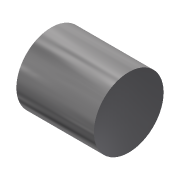
# Autodesk Inventor part: おもり
Saved by Autodesk Inventor 2013 (Build 170138000, 138)
## iProperties
Created: 2013-12-16
Part Number: おもり
Material: ステンレス鋼
Document SubType Name: Modeling
Designer: victor
Mass: 642.534 g
Surface Area: 102.494 cm^2
Volume: 79.5216 cm^3
Density: 8.08 g/cm^3
Author: victor
Autodesk Inventor part; units mm, degrees
ref_plane "YZ Plane" through (0, 0, 0) normal (1, 0, 0) x (0, 1, 0)
ref_plane "XZ Plane" through (0, 0, 0) normal (0, 1, 0) x (-1, 0, 0)
ref_plane "XY Plane" through (0, 0, 0) normal (0, 0, 1) x (1, 0, 0)
sketch "スケッチ1" plane through (0, 0, 0) normal (1, 0, 0) x (0, 1, 0)
  circle A0 centre (4.4898, -7.589) radius 22.5
  point P0 (0, 0)
  dimension "d0" = 45
  dimension "d0" = 45
  constraints: 1 centre point
  measures "d0" diameter of A0
extrude "押し出し1" add sketch "スケッチ1" along normal blind 50
